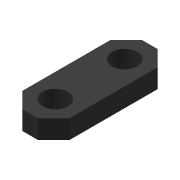
# Autodesk Inventor part: Link
Saved by Autodesk Inventor 2022 Beta2 (Build 260130000, 130) ContinuousBuild 0
## iProperties
Created: 2006-01-31
Part Number: Link
Document SubType Name: Modeling
Designer: landrews
Density: 1 g/cm^3
Material: Generic
Appearance: Generic
Author: landrews
Autodesk Inventor part; units mm, degrees
ref_plane "YZ Plane" through (0, 0, 0) normal (1, 0, 0) x (0, 1, 0)
ref_plane "XZ Plane" through (0, 0, 0) normal (0, 1, 0) x (-1, 0, 0)
ref_plane "XY Plane" through (0, 0, 0) normal (0, 0, 1) x (1, 0, 0)
sketch "Sketch1" plane through (0, 0, 0) normal (0, 0, 1) x (1, 0, 0)
  line L0 (-9, 0) -> (12, 0) projected
  line L1 (0, 30.4) -> (0, -22.8) projected
  line L2 (-2.5, 19) -> (2.5, 19)
  line L3 (2.5, 19) -> (7.5, 14)
  line L4 (7.5, 14) -> (7.5, -14)
  line L5 (7.5, -14) -> (2.5, -19)
  line L6 (2.5, -19) -> (-2.5, -19)
  line L7 (-2.5, -19) -> (-7.5, -14)
  line L8 (-7.5, -14) -> (-7.5, 14)
  line L9 (-7.5, 14) -> (-2.5, 19)
  dimension "d0" = 5
  dimension "d1" = 38
  dimension "d2" = 5
  dimension "d3" = 45
  dimension "d5" = 45
  dimension "d6" = 45
  dimension "d7" = 5
  dimension "d8" = 15
  dimension "d10" = 5
  constraints: 16 end point, 3 perpendicular, 2 parallel, 2 other
  measures "d0" horizontal distance of L2.end L3.end
  measures "d1" distance between parallel lines of L6 L2
  measures "d2" horizontal distance of L4.end L5.end
  measures "d3" angle of L6 L5
  measures "d5" angle of L2 L9
  measures "d6" angle of L3 L2
  measures "d7" horizontal distance of L6.end L7.end
  measures "d8" distance between parallel lines of L4 L8
  measures "d10" horizontal distance of L8.end L2.start
extrude "Extrusion1" add sketch "Sketch1" along normal blind 6
sketch "Sketch2" plane through (0, 0, 6) normal (0, 0, 1) x (1, 0, 0)
  line L0 (-2.5, 19) -> (2.5, 19) projected
  line L1 (2.5, -19) -> (-2.5, -19) projected
  line L2 (0, 30.4) -> (0, -22.8) projected
  point P0 (0, 11)
  point P1 (0, -11)
  dimension "d13" = 8
  dimension "d14" = 8
  constraints: 2 point on line
  measures "d13" distance from line of L0 point (0, 11)
  measures "d14" distance from line of L1 point (0, -11)
hole "Hole1" at (0, 11, 6) at (0, -11, 6) direction (0, 0, -1) diameter 8 end through all
body "Solid1"
